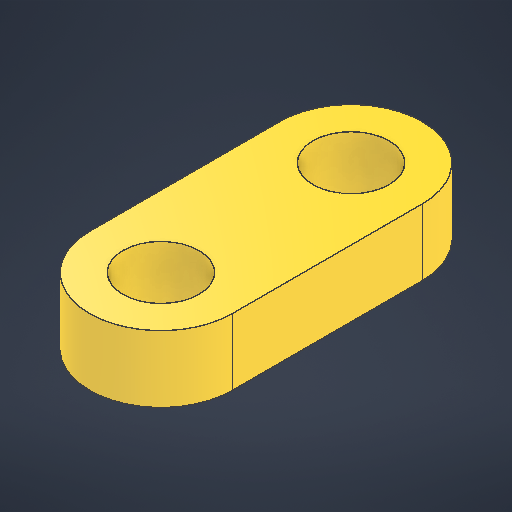
# Autodesk Inventor part: piulita
Saved by Autodesk Inventor 2026.1 (Build 301233000, 233)
## iProperties
Created: 2026-05-19
Part Number: piulita
Material: Generic
Document SubType Name: Modeling
Designer: emanuel
Density: 1 g/cm^3
Appearance: Default
Author: emanuel
Autodesk Inventor part; units mm, degrees
ref_plane "YZ Plane" through (0, 0, 0) normal (1, 0, 0) x (0, 1, 0)
ref_plane "XZ Plane" through (0, 0, 0) normal (0, 1, 0) x (-1, 0, 0)
ref_plane "XY Plane" through (0, 0, 0) normal (0, 0, 1) x (1, 0, 0)
sketch "Sketch1" plane through (0, 0, 0) normal (0, 1, 0) x (-1, 0, 0)
  line L0 (0, 5) -> (0, -5)
  circle A0 centre (0, 5) radius 2
  circle A1 centre (0, -5) radius 2
  line L1 (0, 5) -> (0, -5) construction
  line L2 (-3.75, 5) -> (-3.75, -5)
  line L3 (3.75, -5) -> (3.75, 5)
  arc A2 (3.75, 5) -> (-3.75, 5) centre (0, 5) ccw
  arc A3 (-3.75, -5) -> (3.75, -5) centre (0, -5) ccw
  point P0 (0, 0)
  point P1 (0, 0)
  dimension "d0" = 10
  dimension "d1" = 4
  dimension "d2" = 4
  dimension "d3" = 7.5
  constraints: 10 end point, 4 centre point, 4 point on circle, 4 tangent, 2 coincident, 2 equal length, 2 midpoint, 1 vertical
  measures "d0" distance of L0.start L0.end
  measures "d1" diameter of A0
  measures "d2" diameter of A1
  measures "d3" diameter of A3
extrude "Extrusion1" add sketch "Sketch1" along normal blind 3.5
body "Solid1"
